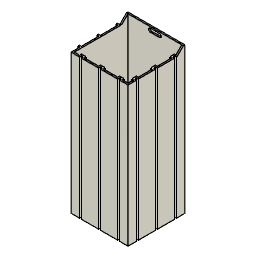
Hardcase_Gridfinity_Bin No Lid (Autodesk Fusion 360 design; units mm, degrees)
part number: 2026-06-11-11-25-00-932
Autodesk Fusion 360 part; units mm, degrees
sketch "Body" plane through (0, 0, 0) normal (0, 1, 0) x (1, 0, 0)
  line L0 (-22.5, -22.5) -> (22.5, -22.5)
  line L1 (22.5, -22.5) -> (22.5, 22.5)
  line L2 (22.5, 22.5) -> (-22.5, 22.5)
  line L3 (-22.5, 22.5) -> (-22.5, -22.5)
  line L4 (-22.5, -22.5) -> (22.5, 22.5) construction
  line L5 (22.5, -22.5) -> (-22.5, 22.5) construction
  line L6 (22.4, 22.4) -> (-22.4, 22.4)
  line L7 (-22.4, 22.4) -> (-22.4, -22.4)
  line L8 (-22.4, -22.4) -> (22.4, -22.4)
  line L9 (22.4, -22.4) -> (22.4, 22.4)
  line L10 (-21.2, 21.2) -> (-21.2, -21.2)
  line L11 (-21.2, -21.2) -> (21.2, -21.2)
  line L12 (21.2, -21.2) -> (21.2, 21.2)
  line L13 (21.2, 21.2) -> (-21.2, 21.2)
  line L14 (-22.5, -22.5) -> (-15.7, -22.5) construction
  line L15 (-15.7, -22.5) -> (-15.7, -22.4) construction
  line L16 (-15.7, -22.4) -> (-22.5, -22.4) construction
  line L17 (-22.5, -22.4) -> (-22.5, -22.5) construction
  line L18 (-22.5, -22.5) -> (-22.4, -22.5) construction
  line L19 (-22.4, -22.5) -> (-22.4, -14.4) construction
  line L20 (-22.4, -14.4) -> (-22.5, -14.4) construction
  line L21 (-22.5, -14.4) -> (-22.5, -22.5) construction
  line L22 (-22.4, -14.4) -> (-23.9, -14.4)
  line L23 (-23.9, -14.4) -> (-23.9, -15.6)
  line L24 (-23.9, -15.6) -> (-22.4, -15.6)
  line L25 (-22.4, -15.6) -> (-22.4, -14.4)
  line L26 (-15.7, -22.4) -> (-14.3, -22.4)
  line L27 (-14.3, -22.4) -> (-14.3, -20.9)
  line L28 (-14.3, -20.9) -> (-15.7, -20.9)
  line L29 (-15.7, -20.9) -> (-15.7, -22.4)
  line L30 (-13.1, -22.4) -> (-13.1, -19.7)
  line L31 (-13.1, -19.7) -> (-16.9, -19.7)
  line L32 (-16.9, -19.7) -> (-16.9, -22.4)
  line L33 (0, -22.5) -> (0, -28) construction
  line L34 (-22.5, 0) -> (-38.981, 0) construction
  line L35 (-22.5, 22.5) -> (-14.4, 22.5) construction
  line L36 (-14.4, 22.5) -> (-14.4, 22.4) construction
  line L37 (-14.4, 22.4) -> (-22.5, 22.4) construction
  line L38 (-22.5, 22.4) -> (-22.5, 22.5) construction
  line L39 (22.5, -22.5) -> (22.4, -22.5) construction
  line L40 (22.4, -22.5) -> (22.4, -15.7) construction
  line L41 (22.4, -15.7) -> (22.5, -15.7) construction
  line L42 (22.5, -15.7) -> (22.5, -22.5) construction
  line L43 (-14.4, 22.4) -> (-15.6, 22.4)
  line L44 (-15.6, 22.4) -> (-15.6, 23.9)
  line L45 (-15.6, 23.9) -> (-14.4, 23.9)
  line L46 (-14.4, 23.9) -> (-14.4, 22.4)
  line L47 (22.4, 16.2) -> (-22.4, 16.2)
  line L48 (22.4, -15.7) -> (20.9, -15.7)
  line L49 (20.9, -15.7) -> (20.9, -14.3)
  line L50 (20.9, -14.3) -> (22.4, -14.3)
  line L51 (22.4, -14.3) -> (22.4, -15.7)
  line L52 (22.4, -16.9) -> (19.7, -16.9)
  line L53 (19.7, -16.9) -> (19.7, -13.1)
  line L54 (19.7, -13.1) -> (22.4, -13.1)
  dimension "d39" = 45
  dimension "d40" = 45
  dimension "d43" = 6.8
  dimension "d44" = 0.1
  dimension "d45" = 0.1
  dimension "d46" = 8.1
  dimension "d47" = 1.5
  dimension "d48" = 1.2
  dimension "d49" = 1.4
  dimension "d50" = 1.5
  dimension "d51" = 1.2
  dimension "d66" = 8.1
  dimension "d67" = 0.1
  dimension "d70" = 0.1
  dimension "d71" = 6.8
  dimension "d81" = 1.2
  dimension "d82" = 1.5
  dimension "d196" = 1.5
  dimension "d197" = 1.4
  constraint horizontal L0
  constraint perpendicular L0 L1
  constraint parallel L0 L2
  constraint parallel L1 L3
  constraint coincident L4 origin
  constraint coincident L5 origin
  constraint horizontal L14
  constraint vertical L15
  constraint horizontal L16
  constraint vertical L17
  constraint horizontal L18
  constraint vertical L19
  constraint horizontal L20
  constraint vertical L21
  constraint horizontal L22
  constraint vertical L23
  constraint horizontal L24
  constraint vertical L25
  constraint horizontal L26
  constraint vertical L27
  constraint horizontal L28
  constraint vertical L29
  constraint coincident L8 L32.end
  constraint coincident L8 L30.start
  constraint midpoint L0 L33.start
  constraint perpendicular L0 L33
  constraint midpoint L3 L34.start
  constraint perpendicular L3 L34
  constraint horizontal L35
  constraint vertical L36
  constraint horizontal L37
  constraint vertical L38
  constraint horizontal L39
  constraint vertical L40
  constraint horizontal L41
  constraint vertical L42
  constraint horizontal L43
  constraint vertical L44
  constraint horizontal L45
  constraint vertical L46
  constraint coincident L7 L47.end
  constraint coincident L9 L47.start
  constraint horizontal L48
  constraint vertical L49
  constraint horizontal L50
  constraint vertical L51
  constraint coincident L9 L54.end
  constraint coincident L40 L52.start
  measures "d39" distance of L1.end L2.end
  measures "d40" distance of L0.end L1.end
  measures "d43" distance of L0.start L14.end
  measures "d44" distance of L0.start L16.end
  measures "d45" distance of L0.start L18.end
  measures "d46" distance of L0.start L20.end
  measures "d47" distance of L19.end L22.end
  measures "d48" distance of L19.end L24.end
  measures "d49" distance of L15.end L26.end
  measures "d50" distance of L15.end L28.end
  measures "d66" distance of L2.end L35.end
  measures "d67" distance of L2.end L37.end
  measures "d70" distance of L0.end L39.end
  measures "d71" distance of L0.end L41.end
  measures "d81" distance of L36.end L43.end
  measures "d82" distance of L36.end L45.end
  measures "d196" distance of L40.end L48.end
  measures "d197" distance of L40.end L50.end
extrude "Extrude1" add sketch "Body" along normal blind 110 contours L7 L8 L10 L11 L25 L32 L47 | L6 L7 L9 L10 L12 L13 L43 L47 | L8 L11 L29 L32 | L8 L11 L26 L27 L29 | L9 L12 L47 L54 | L8 L11 L27 L30 | L9 L12 L50 L54 | L8 L9 L11 L12 L30 L52 | L9 L12 L48 L50 L51 | L9 L12 L48 L52 makes body 1
ref_plane "WorkPlane3" through (0, 55, 0) normal (0, 1, 0) x (0, 0, 1)
sketch "Floor" plane through (0, 55, 0) normal (0, 1, 0) x (1, 0, 0)
  line L0 (-22.5, -22.5) -> (22.5, -22.5)
  line L1 (22.5, -22.5) -> (22.5, 22.5)
  line L2 (22.5, 22.5) -> (-22.5, 22.5)
  line L3 (-22.5, 22.5) -> (-22.5, -22.5)
  line L4 (-22.5, -22.5) -> (22.5, 22.5) construction
  line L5 (22.5, -22.5) -> (-22.5, 22.5) construction
  line L6 (-22.4, 22.4) -> (-22.4, -22.4)
  line L7 (-22.4, -22.4) -> (22.4, -22.4)
  line L8 (22.4, -22.4) -> (22.4, 22.4)
  line L9 (22.4, 22.4) -> (-22.4, 22.4)
  line L10 (-21.3, 21.3) -> (-21.3, -21.3)
  line L11 (-21.3, -21.3) -> (21.3, -21.3)
  line L12 (21.3, -21.3) -> (21.3, 21.3)
  line L13 (21.3, 21.3) -> (-21.3, 21.3)
  line L14 (0, 21.3) -> (-20.6, 21.3) construction
  line L15 (-20.6, 21.3) -> (-20.6, 21.1) construction
  line L16 (-20.6, 21.1) -> (0, 21.1) construction
  line L17 (0, 21.1) -> (0, 21.3) construction
  line L18 (0, 21.3) -> (19.1, 21.3) construction
  line L19 (19.1, 21.3) -> (19.1, 21.1) construction
  line L20 (19.1, 21.1) -> (0, 21.1) construction
  line L21 (0, 21.1) -> (0, 21.3) construction
  line L22 (-20.6, 21.1) -> (-21.7, 21.1)
  line L23 (-21.7, 21.1) -> (-21.7, 20.1)
  line L24 (-21.7, 20.1) -> (-20.6, 20.1)
  line L25 (-20.6, 20.1) -> (-20.6, 21.1)
  line L26 (-21.7, 20.1) -> (-20.6, 21.1)
  line L27 (19.1, 21.1) -> (20.2, 21.1)
  line L28 (20.2, 21.1) -> (20.2, 20.1)
  line L29 (20.2, 20.1) -> (19.1, 20.1)
  line L30 (19.1, 20.1) -> (19.1, 21.1)
  line L31 (19.1, 21.1) -> (20.2, 20.1)
  dimension "d219" = 45
  dimension "d220" = 45
  dimension "d243" = 20.6
  dimension "d244" = 0.2
  dimension "d245" = 19.1
  dimension "d246" = 0.2
  dimension "d247" = 1.1
  dimension "d248" = 1
  dimension "d249" = 1.1
  dimension "d250" = 1
  constraint horizontal L0
  constraint perpendicular L0 L1
  constraint parallel L0 L2
  constraint parallel L1 L3
  constraint coincident L4 origin
  constraint coincident L5 origin
  constraint horizontal L14
  constraint vertical L15
  constraint horizontal L16
  constraint vertical L17
  constraint midpoint L13 L14.start
  constraint horizontal L18
  constraint vertical L19
  constraint horizontal L20
  constraint vertical L21
  constraint horizontal L22
  constraint vertical L23
  constraint horizontal L24
  constraint vertical L25
  constraint horizontal L27
  constraint vertical L28
  constraint horizontal L29
  constraint vertical L30
  measures "d219" distance of L1.end L2.end
  measures "d220" distance of L0.end L1.end
  measures "d243" distance of L14.start L14.end
  measures "d244" distance of L14.start L16.end
  measures "d245" distance of L14.start L18.end
  measures "d246" distance of L14.start L16.end
  measures "d247" distance of L15.end L22.end
  measures "d248" distance of L15.end L24.end
  measures "d249" distance of L19.end L27.end
  measures "d250" distance of L19.end L29.end
extrude "Extrude19" add sketch "Floor" along normal blind 1 from surface at -55 contours L10 L11 L12 L13 L22 L24 L25 | L10 L22 L26 | L10 L24 L25 L26 | L29 L30 L31 | L27 L28 L31 bodies 1
extrude "Extrude3" add sketch "Body" along normal blind 110 contours L8 L11 L29 L32 | L11 L27 L28 L29 L30 L31 L32 | L8 L11 L27 L30 bodies 1
extrude "Extrude4" cut sketch "Body" along normal blind 110 contours L8 L11 L26 L27 L29 | L11 L27 L28 L29 bodies 1
extrude "Extrude8" add sketch "Body" along normal blind 110 contours L2 L6 L43 L44 L46 | L2 L44 L45 L46 bodies 1
extrude "Extrude5" add sketch "Body" along normal blind 110 contours L3 L22 L23 L24 | L3 L7 L22 L24 L25 bodies 1
extrude "Extrude6" add sketch "Body" along normal blind 110 contours L9 L12 L50 L54 | L12 L48 L49 L50 L52 L53 L54 | L9 L12 L48 L52 bodies 1
extrude "Extrude7" cut sketch "Body" along normal blind 110 contours L9 L12 L48 L50 L51 | L12 L48 L49 L50 bodies 1
pattern_linear "R-Pattern1" count 3 spacing 15 along (1, 0, 0) of "Extrude3", "Extrude4", "Extrude8"
pattern_linear "R-Pattern2" count 3 spacing 15 along (0, 0, -1) of "Extrude5", "Extrude6", "Extrude7"
extrude "Extrude15" add sketch "Body" along normal blind 5 from surface at 110 contours L6 L7 L9 L10 L12 L13 L43 L47 bodies 1
chamfer "Chamfer1" distance 5 angle 45 2 edges at (21.8, 115, -16.2) (-21.8, 115, -16.2) on bodies 1
sketch "Pull Tab Hole" plane through (0, 0, 0) normal (0, 0, 1) x (1, 0, 0)
  line L0 (0, 0) -> (0, 110) construction
  line L1 (0, 110) -> (0, 112.5) construction
  line L2 (3.726, 113.8) -> (-3.726, 113.8)
  line L3 (-5, 112.526) -> (-5, 112.474)
  line L4 (-3.726, 111.2) -> (3.726, 111.2)
  line L5 (5, 112.474) -> (5, 112.526)
  line L6 (5, 113.8) -> (-5, 111.2) construction
  line L7 (-5, 113.8) -> (5, 111.2) construction
  arc A0 (-5, 112.474) -> (-3.726, 111.2) centre (-3.726, 112.474) ccw
  arc A1 (-3.726, 113.8) -> (-5, 112.526) centre (-3.726, 112.526) ccw
  arc A2 (5, 112.526) -> (3.726, 113.8) centre (3.726, 112.526) ccw
  arc A3 (3.726, 111.2) -> (5, 112.474) centre (3.726, 112.474) ccw
  point P0 (0, 112.5)
  dimension "d180" = 110
  dimension "d181" = 2.5
  dimension "d182" = 10
  dimension "d183" = 2.6
  dimension "d184" = 1.274
  constraint coincident L0.start origin
  constraint vertical L0
  constraint parallel L0 L1
  constraint horizontal L2
  constraint perpendicular L2 L3
  constraint parallel L2 L4
  constraint parallel L3 L5
  constraint coincident L6 P0
  constraint coincident L7 P0
  constraint coincident P0 L1.end
  constraint coincident L6.end L3
  constraint coincident L6.end L4
  constraint tangent L3 A0
  constraint tangent L4 A0
  constraint coincident L7.start L3
  constraint coincident L7.start L2
  constraint tangent L3 A1
  constraint tangent L2 A1
  constraint equal A0 A1
  constraint coincident L6.start L2
  constraint coincident L6.start L5
  constraint tangent L2 A2
  constraint tangent L5 A2
  constraint equal A0 A2
  constraint coincident L7.end L4
  constraint coincident L7.end L5
  constraint tangent L4 A3
  constraint tangent L5 A3
  constraint equal A0 A3
  measures "d180" distance of L0.start L0.end
  measures "d181" distance of L0.end P0
  measures "d182" distance of L6.end L7.end
  measures "d183" distance of L7.start L6.end
  measures "d184" radius of A0
extrude "Extrude16" cut sketch "Pull Tab Hole" against normal blind 45 bodies 1
copy_body "Body->Comp3" bodies 1 removing the originals makes body 2 in component "Body"
component "Body" placed x (1, 0, 0) y (0, 1, 0) z (0, 0, 1) at (0, 0, 0)
equation "GRID_SPACING = 15 mm"
equation "WALL_THICK = 1.2 mm"
equation "WALL_BUMP = 1.5 mm"
equation "CLEAR = 0.1 mm"
equation "LENGTH_MODULE_NUMBER = 3"
equation "WIDTH_MODULE_NUMBER = 3"
equation "OVERALL_HT = 110 mm"
equation "FLOOR_THICK = 1 mm"
equation "d31 = OVERALL_HT"
equation "d35 = OVERALL_HT"
equation "d37 = OVERALL_HT"
equation "d39 = LENGTH_MODULE_NUMBER * GRID_SPACING"
equation "d40 = WIDTH_MODULE_NUMBER * GRID_SPACING"
equation "d41 = -CLEAR"
equation "d42 = -WALL_THICK"
equation "d43 = GRID_SPACING / 2 - WALL_THICK / 2 - CLEAR"
equation "d44 = CLEAR"
equation "d45 = CLEAR"
equation "d46 = GRID_SPACING / 2 + WALL_THICK / 2"
equation "d47 = WALL_BUMP"
equation "d48 = WALL_THICK"
equation "d49 = WALL_THICK + CLEAR * 2"
equation "d50 = WALL_BUMP"
equation "d51 = WALL_THICK"
equation "d52 = LENGTH_MODULE_NUMBER"
equation "d54 = GRID_SPACING"
equation "d56 = OVERALL_HT"
equation "d58 = WIDTH_MODULE_NUMBER"
equation "d60 = GRID_SPACING"
equation "d66 = GRID_SPACING / 2 + WALL_THICK / 2"
equation "d67 = CLEAR"
equation "d70 = CLEAR"
equation "d71 = GRID_SPACING / 2 - WALL_THICK / 2 - CLEAR"
equation "d75 = OVERALL_HT"
equation "d77 = OVERALL_HT"
equation "d79 = OVERALL_HT"
equation "d81 = WALL_THICK"
equation "d82 = WALL_BUMP"
equation "LID_THICK = 3 mm"
equation "LID_TOP_OFFSET = 1 mm"
equation "LID_LOCK_LENGTH = 8 mm"
equation "LID_PULL_WIDTH = 8 mm"
equation "LID_PULL_HT = 1 mm"
equation "LID_PULL_FRONT_OFFSET = 3 mm"
equation "PULL_TAB_WIDTH = PULL_TAB_HT + WALL_THICK"
equation "d172 = -PULL_TAB_WIDTH"
equation "d173 = OVERALL_HT"
equation "d174 = PULL_TAB_HT"
equation "PULL_TAB_HT = 5 mm"
equation "d179 = PULL_TAB_HT"
equation "d180 = OVERALL_HT"
equation "d181 = PULL_TAB_HT / 2"
equation "d182 = PULL_HOLE_LENGTH"
equation "d183 = PULL_TAB_HT - WALL_THICK * 2"
equation "d184 = ( PULL_TAB_HT - WALL_THICK * 2 ) * 0.49"
equation "d185 = -WIDTH_MODULE_NUMBER * GRID_SPACING"
equation "PULL_HOLE_LENGTH = 10 mm"
equation "d196 = WALL_BUMP"
equation "d197 = WALL_THICK + CLEAR * 2"
equation "d198 = -WALL_THICK"
equation "d200 = OVERALL_HT / 2"
equation "d219 = LENGTH_MODULE_NUMBER * GRID_SPACING"
equation "d220 = WIDTH_MODULE_NUMBER * GRID_SPACING"
equation "d221 = -CLEAR"
equation "d222 = -WALL_THICK"
equation "d223 = FLOOR_THICK"
equation "LID_CLEAR = 0.1 mm"
equation "CHAMFER_LENGTH = 0.5 mm"
equation "CHAMFER_WIDTH = 1 mm"
equation "d243 = ( GRID_SPACING * LENGTH_MODULE_NUMBER ) / 2 - WALL_THICK - CLEAR - LID_CLEAR - CHAMFER_LENGTH"
equation "d244 = LID_CLEAR + CLEAR"
equation "d245 = ( LENGTH_MODULE_NUMBER * GRID_SPACING ) / 2 - WALL_BUMP - WALL_THICK - CLEAR - LID_CLEAR - CHAMFER_LENGTH"
equation "d246 = LID_CLEAR + CLEAR"
equation "d247 = WALL_THICK / 2 + CHAMFER_LENGTH"
equation "d248 = CHAMFER_WIDTH"
equation "d249 = WALL_THICK / 2 + CHAMFER_LENGTH"
equation "d250 = CHAMFER_WIDTH"
equation "d253 = -OVERALL_HT / 2"
equation "LID_LOCK_OFFSET = 0.1 mm"
named bodies: "Body"
